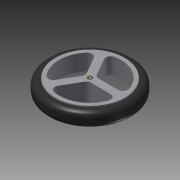
# Autodesk Inventor part: n2_miniWheel
Saved by Autodesk Inventor 2015 (Build 190159000, 159)
## iProperties
Created: 2017-10-15
Part Number: n2_miniWheel
Material: Generic
Document SubType Name: Modeling
Designer: tlsru
Density: 1 g/cm^3
Appearance: Default
Author: tlsru
Autodesk Inventor part; units mm, degrees
ref_plane "YZ Plane" through (0, 0, 0) normal (1, 0, 0) x (0, 1, 0)
ref_plane "XZ Plane" through (0, 0, 0) normal (0, 1, 0) x (-1, 0, 0)
ref_plane "XY Plane" through (0, 0, 0) normal (0, 0, 1) x (1, 0, 0)
sketch "스케치1" plane through (0, 0, 0) normal (0, 0, 1) x (1, 0, 0)
  circle A0 centre (0, 0) radius 4.1
  circle A1 centre (0, 0) radius 1 projected
  dimension "d0" = 8.2
  constraints: 1 centre point, 1 coincident
  measures "d0" diameter of A0
extrude "돌출1" add sketch "스케치1" along normal blind 8.62
sketch "스케치2" plane through (0, 0, 8.62) normal (0, 0, 1) x (1, 0, 0)
  circle A0 centre (0, 0) radius 17
  circle A1 centre (0, 0) radius 4.1 projected
  dimension "d3" = 34
  constraints: 1 centre point, 1 coincident
  measures "d3" diameter of A0
extrude "돌출2" add sketch "스케치2" against normal blind 6.6
sketch "스케치3" plane through (0, 0, 8.62) normal (0, 0, 1) x (1, 0, 0)
  point P0 (0, 0)
sketch "스케치4" plane through (0, 0, 8.62) normal (0, 0, 1) x (1, 0, 0)
  circle A0 centre (0, 0) radius 17 projected
  circle A1 centre (0, 0) radius 1 projected
  circle A2 centre (0, 0) radius 14
  dimension "d6" = 3
  constraints: 1 centre point
  measures "d6" radial gap between concentric circles of A0 A2
extrude "돌출3" cut sketch "스케치4" against normal blind 0.5 contours A0
sketch "스케치5" plane through (0, 0, 2.02) normal (0, 0, -1) x (-1, 0, 0)
  circle A0 centre (0, 0) radius 4.1 projected
  circle A1 centre (0, 0) radius 17 projected
  circle A2 centre (0, 0) radius 14 projected
extrude "돌출4" cut sketch "스케치5" against normal blind 0.5 contours A1
fillet "모깎기1" radius 2 2 edges at (-17, 0, 2.52) (-17, 0, 8.12)
sketch "스케치6" plane through (0, 0, 8.62) normal (0, 0, 1) x (1, 0, 0)
  circle A0 centre (0, 0) radius 14 projected
  circle A1 centre (0, 0) radius 1 projected
  circle A2 centre (0, 0) radius 14
  circle A3 centre (0, 0) radius 14 projected
  line L0 (0, 0) -> (1, 0) construction
  line L1 (0, 0) -> (-0.5, -0.866)
  line L2 (2.026, -1.5128) -> (9.8898, -1.5625)
  line L3 (0.866, -1.5) -> (0.8629, -1.5055)
  line L4 (-2.3094, -1) -> (-6.2488, -7.8232)
  line L5 (13.9097, -1.5879) -> (13.9902, -1.5884)
  line L6 (0.296, 2.4873) -> (-3.6507, 9.3232)
  line L7 (-2.3094, 1) -> (-6.2488, 7.8232)
  line L8 (-8.2587, 11.3046) -> (-8.299, 11.3744)
  line L9 (-5.6607, 12.8046) -> (-5.701, 12.8744)
  arc A4 (-2.2841, -12.2895) -> (11.7585, -4.2411) centre (0, 0) ccw
  line L10 (0, 0) -> (1, -0.0063)
  line L11 (0.2813, -2.5128) -> (-3.6507, -9.3232)
  line L12 (-5.6607, -12.8046) -> (-5.701, -12.8744)
  line L13 (0, 0) -> (-0.5, 0.866)
  line L14 (2.0154, 1.4873) -> (9.9088, 1.4374)
  line L15 (13.9286, 1.412) -> (14.0092, 1.4115)
  arc A5 (11.8112, 4.0921) -> (-2.2841, 12.2895) centre (0, 0) ccw
  arc A6 (-9.501, 8.1229) -> (-9.501, -8.1229) centre (0, 0) ccw
  line L16 (0, 0) -> (1, 0) construction
  arc A7 (9.9088, 1.4374) -> (11.8112, 4.0921) centre (9.9214, 3.4374) ccw
  arc A8 (-2.2841, 12.2895) -> (-3.6507, 9.3232) centre (-1.9187, 10.3232) ccw
  arc A9 (0.296, 2.4873) -> (2.0154, 1.4873) centre (2.0281, 3.4873) ccw
  arc A10 (2.026, -1.5128) -> (0.2813, -2.5128) centre (2.0133, -3.5128) ccw
  arc A11 (11.7585, -4.2411) -> (9.8898, -1.5625) centre (9.8772, -3.5625) ccw
  arc A12 (-3.6507, -9.3232) -> (-2.2841, -12.2895) centre (-1.9187, -10.3232) ccw
  arc A13 (-9.501, -8.1229) -> (-6.2488, -7.8232) centre (-7.9808, -6.8232) ccw
  arc A14 (-6.2488, 7.8232) -> (-9.501, 8.1229) centre (-7.9808, 6.8232) ccw
  arc A15 (-2.3094, -1) -> (-2.3094, 1) centre (-4.0415, 0) ccw
  point P0 (12.4189, 1.4215)
  point P1 (12.3999, -1.5784)
  point P2 (-4.9058, -11.4971)
  point P3 (-7.5039, -9.9971)
  point P4 (-7.5039, 9.9971)
  point P5 (-4.9058, 11.4971)
  dimension "d26" = 1.5
  dimension "d28" = 1.5
  dimension "d29" = 2
  constraints: 39 point on circle, 34 end point, 18 tangent, 13 centre point, 12 parallel, 8 equal radius, 8 point on line, 2 horizontal, 1 coincident
  measures "d26" distance between parallel lines of L1 L3
  measures "d28" distance between parallel lines of L1 L4
  measures "d29" radius of A7
extrude "돌출5" cut sketch "스케치6" against normal up to next contours L2 A11 A4 A12 L11 A10 | L4 A13 A6 A14 L7 A15 | L6 A8 A5 A7 L14 A9
